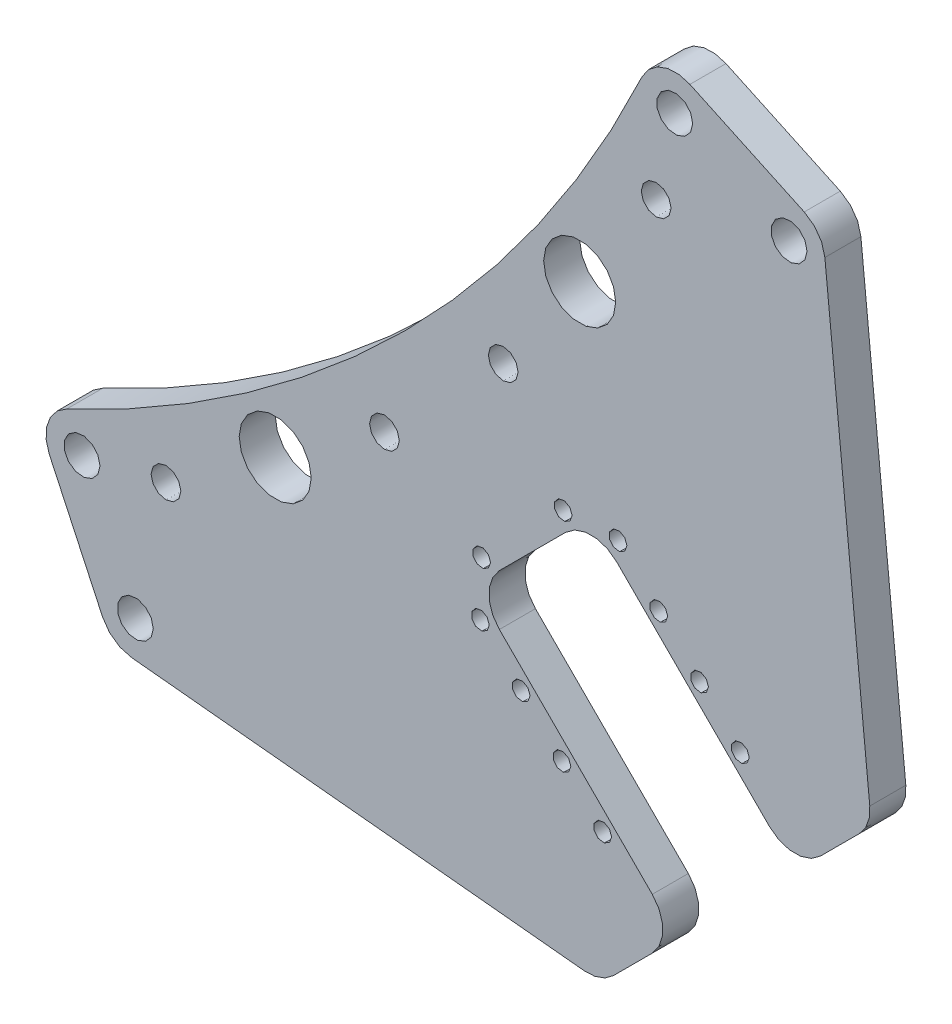
# Autodesk Inventor part: motorplate
Saved by Autodesk Inventor 2015 (Build 190159000, 159)
## iProperties
Created: 2015-02-25
Part Number: motorplate
Material: Generic
Document SubType Name: Modeling
Designer: janov_000
Density: 1 g/cm^3
Appearance: Aluminum - Flat
Author: janov_000
Autodesk Inventor part; units mm, degrees
ref_plane "YZ Plane" through (0, 0, 0) normal (1, 0, 0) x (0, 1, 0)
ref_plane "XZ Plane" through (0, 0, 0) normal (0, 1, 0) x (-1, 0, 0)
ref_plane "XY Plane" through (0, 0, 0) normal (0, 0, 1) x (1, 0, 0)
sketch "Sketch1" plane through (0, 0, 0) normal (0, 0, 1) x (1, 0, 0)
  circle A0 centre (-3.6979, 7.9302) radius 2.5 construction
  circle A1 centre (3.6979, -7.9302) radius 2.5 construction
  line L0 (-8.2294, 5.8171) -> (-0.8336, -10.0433) construction
  arc A2 (-0.8336, -10.0433) -> (8.2294, -5.8171) centre (3.6979, -7.9302) ccw construction
  line L1 (8.2294, -5.8171) -> (0.8336, 10.0433) construction
  arc A3 (0.8336, 10.0433) -> (-8.2294, 5.8171) centre (-3.6979, 7.9302) ccw construction
  circle A4 centre (78.5293, 90.1574) radius 2.5 construction
  circle A5 centre (94.3897, 82.7616) radius 2.5 construction
  line L2 (76.4162, 85.6259) -> (92.2766, 78.2301) construction
  arc A6 (92.2766, 78.2301) -> (96.5028, 87.2931) centre (94.3897, 82.7616) ccw construction
  line L3 (96.5028, 87.2931) -> (80.6424, 94.689) construction
  arc A7 (80.6424, 94.689) -> (76.4162, 85.6259) centre (78.5293, 90.1574) ccw construction
  circle A8 centre (-75.543, 162.0025) radius 75 construction
  line L4 (112.457, 50.5739) -> (112.457, -27.9975) construction
  line L5 (107.457, -32.9975) -> (39.927, -32.9975) construction
  line L6 (-75.543, 162.0025) -> (58.8073, 27.6522) construction
  line L7 (54.2111, 23.056) -> (63.4035, 32.2484)
  line L8 (70.4745, 32.2484) -> (91.6877, 11.0352)
  line L9 (54.2111, 15.985) -> (75.4243, -5.2282)
  line L10 (75.4243, -12.2993) -> (70.027, -17.6966)
  line L11 (98.7588, 11.0352) -> (104.1561, 16.4325)
  line L12 (-0.8336, -10.0433) -> (-8.2294, 5.8171)
  line L13 (80.6424, 94.689) -> (96.5028, 87.2931)
  arc A9 (-5.811, 12.4617) -> (73.9978, 92.2705) centre (-75.543, 162.0025) ccw
  line L14 (-3.6979, 7.9302) -> (3.6979, -7.9302) construction
  line L15 (78.5293, 90.1574) -> (94.3897, 82.7616) construction
  line L16 (65.9977, -19.1366) -> (3.2042, -12.9058)
  line L17 (105.5961, 20.4618) -> (99.3653, 83.2553)
  arc A10 (75.4243, -12.2993) -> (75.4243, -5.2282) centre (71.8887, -8.7638) ccw
  arc A11 (54.2111, 23.056) -> (54.2111, 15.985) centre (57.7466, 19.5205) ccw
  arc A12 (70.4745, 32.2484) -> (63.4035, 32.2484) centre (66.939, 28.7129) ccw
  arc A13 (91.6877, 11.0352) -> (98.7588, 11.0352) centre (95.2233, 14.5708) ccw
  arc A14 (104.1561, 16.4325) -> (105.5961, 20.4618) centre (100.6206, 19.9681) ccw
  arc A15 (99.3653, 83.2553) -> (96.5028, 87.2931) centre (94.3897, 82.7616) ccw
  arc A16 (80.6424, 94.689) -> (73.9978, 92.2705) centre (78.5293, 90.1574) ccw
  arc A17 (-5.811, 12.4617) -> (-8.2294, 5.8171) centre (-3.6979, 7.9302) ccw
  arc A18 (-0.8336, -10.0433) -> (3.2042, -12.9058) centre (3.6979, -7.9302) ccw
  arc A19 (65.9977, -19.1366) -> (70.027, -17.6966) centre (66.4914, -14.1611) ccw
  point P0 (0, 0)
  point P1 (79.4008, -9.1758)
  point P2 (50.6755, 19.5205)
  point P3 (66.939, 35.784)
  point P4 (95.2233, 7.4997)
  point P5 (78.9598, -8.7638)
  point P6 (68.3532, -19.3704)
  point P7 (105.8299, 18.1063)
  point P8 (0.37, -12.6245)
  point P9 (76.0422, 96.8341)
  point P10 (99.084, 86.0895)
  point P11 (-10.3746, 10.4173)
  point P12 (-4.5315, -2.1131)
  point P13 (88.5726, 90.991)
  dimension "d56" = 190
  dimension "d64" = 23
  dimension "d65" = 40
  dimension "d67" = 165
  dimension "d68" = 15
  dimension "d69" = 15
  dimension "d70" = 20
  dimension "d73" = 5
  constraints: 24 end point, 24 point on circle, 22 tangent, 18 point on line, 11 centre point, 9 equal radius, 6 coincident, 5 midpoint, 5 perpendicular, 2 parallel, 1 collinear
  measures "d56" distance of L6.end L6.start
  measures "d64" distance of point (50.676, 19.521) point (66.939, 35.784)
  measures "d65" distance of point (66.939, 35.784) point (95.223, 7.5)
  measures "d67" radius of A9
  measures "d68" distance of point (78.96, -8.764) point (68.353, -19.37)
  measures "d69" distance of point (95.223, 7.5) point (105.83, 18.106)
  measures "d70" angle of L14 L6
  measures "d73" radius of A10
extrude "Extrusion1" add sketch "Sketch1" along normal blind 5
sketch "Sketch2" plane through (0, 0, 5) normal (0, 0, 1) x (1, 0, 0)
  circle A0 centre (3.6979, -7.9302) radius 2.067 projected
  circle A1 centre (-3.6979, 7.9302) radius 2.067 projected
  circle A2 centre (94.3897, 82.7616) radius 2.067 projected
  circle A3 centre (78.5293, 90.1574) radius 2.067 projected
  point P0 (0, 0)
  constraints: 6 coincident
hole "Hole1" at (78.5293, 90.1574, 5) at (94.3897, 82.7616, 5) at (-3.6979, 7.9302, 5) at (3.6979, -7.9302, 5) direction (0, 0, -1) diameter 5 end through all
sketch "Sketch4" plane through (0, 0, 5) normal (0, 0, 1) x (1, 0, 0)
  circle A0 centre (-3.6979, 7.9302) radius 2.5 projected
  circle A1 centre (78.5293, 90.1574) radius 2.5 projected
  circle A2 centre (94.3897, 82.7616) radius 2.5 projected
  circle A3 centre (3.6979, -7.9302) radius 2.5 projected
  line L0 (-75.543, 162.0025) -> (23.1121, 21.1084) construction
  line L1 (-75.543, 162.0025) -> (-3.6979, 7.9302) construction
  line L2 (78.5293, 90.1574) -> (-75.543, 162.0025) construction
  line L3 (-75.543, 162.0025) -> (65.3511, 63.3474) construction
  circle A4 centre (-75.543, 162.0025) radius 75 projected
  point P0 (0, 0)
  dimension "d27" = 10
  dimension "d28" = 10
  dimension "d71" = 172
  dimension "d72" = 172
  constraints: 8 end point, 5 coincident
  measures "d27" angle of L0 L1
  measures "d28" angle of L2 L3
  measures "d71" distance of L0.start L0.end
  measures "d72" distance of L0.start L3.end
hole "Hole2" at (23.1121, 21.1084, 5) at (65.3511, 63.3474, 5) direction (0, 0, -1) diameter 10 end through all
sketch "Sketch6" plane through (0, 0, 5) normal (0, 0, 1) x (1, 0, 0)
  line L0 (23.1121, 21.1084) -> (7.9578, 10.4972) construction
  line L1 (23.1121, 21.1084) -> (38.2664, 31.7195) construction
  line L2 (23.1121, 21.1084) -> (19.0971, 26.8424) construction
  line L3 (65.3511, 63.3474) -> (54.74, 48.1931) construction
  line L4 (65.3511, 63.3474) -> (75.9623, 78.5017) construction
  line L5 (65.3511, 63.3474) -> (59.6171, 67.3624) construction
  arc A0 (-5.811, 12.4617) -> (73.9978, 92.2705) centre (-75.543, 162.0025) ccw projected
  point P0 (0, 0)
  point P1 (76.0422, 96.8341)
  point P2 (-10.3746, 10.4173)
  dimension "d29" = 18.5
  dimension "d30" = 18.5
  dimension "d38" = 18.5
  dimension "d39" = 18.5
  constraints: 12 end point, 4 coincident, 2 collinear, 2 line through centre, 2 perpendicular
  measures "d29" distance of L0.start L0.end
  measures "d30" distance of L0.start L1.end
  measures "d38" distance of L3.start L3.end
  measures "d39" distance of L3.start L4.end
hole "Hole3" at (7.9578, 10.4972, 5) at (38.2664, 31.7195, 5) at (54.74, 48.1931, 5) at (75.9623, 78.5017, 5) direction (0, 0, -1) diameter 4.134 end through all thread size "M5x0.8" class "6H" standard "ANSI Metric M Profile"
sketch "Sketch7" plane through (0, 0, 5) normal (0, 0, 1) x (1, 0, 0)
  arc A0 (50.3958, 16.2647) -> (52.016, 14.6445) centre (51.5594, 15.8082) ccw projected
  arc A1 (56.0526, 10.6079) -> (57.6728, 8.9877) centre (57.2163, 10.1513) ccw projected
  arc A2 (61.7095, 4.951) -> (63.3297, 3.3308) centre (62.8731, 4.4945) ccw projected
  arc A3 (67.3663, -0.7058) -> (68.9865, -2.326) centre (68.53, -1.1624) ccw projected
  arc A4 (71.815, 34.4435) -> (70.1948, 36.0637) centre (70.6513, 34.9001) ccw projected
  arc A5 (77.4718, 28.7867) -> (75.8516, 30.4069) centre (76.3082, 29.2432) ccw projected
  arc A6 (83.1287, 23.1298) -> (81.5085, 24.75) centre (81.965, 23.5864) ccw projected
  arc A7 (88.7855, 17.473) -> (87.1653, 19.0932) centre (87.6219, 17.9295) ccw projected
  arc A8 (63.5065, 35.8869) -> (61.8863, 34.2668) centre (63.0499, 34.7233) ccw projected
  arc A9 (52.1927, 24.5732) -> (50.5726, 22.953) centre (51.7362, 23.4096) ccw projected
  point P0 (0, 0)
  constraints: 10 coincident
hole "Hole4" at (51.7362, 23.4096, 5) at (63.0499, 34.7233, 5) at (51.5594, 15.8082, 5) at (57.2163, 10.1513, 5) at (62.8731, 4.4945, 5) at (70.6513, 34.9001, 5) at (76.3082, 29.2432, 5) at (81.965, 23.5864, 5) at (68.53, -1.1624, 5) at (87.6219, 17.9295, 5) direction (0, 0, -1) diameter 2.5 end through all
body "Solid1"
